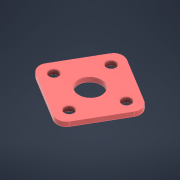
# Autodesk Inventor part: motor bracket n 20
Saved by Autodesk Inventor 2021 (Build 250183000, 183)
## iProperties
Created: 2021-01-01
Part Number: motor bracket n 20
Material: Steel, Mild
Document SubType Name: Modeling
Designer: Vikki
Density: 7.85 g/cm^3
Appearance: Smooth - Red
Author: Vikki
Autodesk Inventor part; units mm, degrees
ref_plane "YZ Plane" through (0, 0, 0) normal (1, 0, 0) x (0, 1, 0)
ref_plane "XZ Plane" through (0, 0, 0) normal (0, 1, 0) x (-1, 0, 0)
ref_plane "XY Plane" through (0, 0, 0) normal (0, 0, 1) x (1, 0, 0)
ref_plane "Work Plane1" through (16.343721, 23.98815, 28.390628) normal (0.0633212, 0.9973467, 0.0359151) x (-0.8897935, 0.0401224, 0.4545962)
sketch "Sketch1" plane through (16.343721, 23.98815, 28.390628) normal (0.0633212, 0.9973467, 0.0359151) x (-0.8897935, 0.0401224, 0.4545962)
  circle A0 centre (9.859, 0) radius 11 construction
  line L0 (12.200549, 7.380964) -> (2.137484, 0.843784)
  line L1 (13.972533, 19.366952) -> (-9.507952, 4.113533)
  line L2 (-9.507952, 4.113533) -> (5.745467, -19.366952)
  line L3 (5.745467, -19.366952) -> (29.225952, -4.113533)
  line L4 (29.225952, -4.113533) -> (13.972533, 19.366952)
  line L5 (13.972533, 19.366952) -> (5.745467, -19.366952) construction
  line L6 (-9.507952, 4.113533) -> (29.225952, -4.113533) construction
  circle A1 centre (9.859, 0) radius 9.5
  circle A2 centre (9.859, 0) radius 9.5
  circle A3 centre (9.859, 0) radius 9.5
  circle A4 centre (9.859, 0) radius 9.5
  point P0 (0.673802, -31.196325)
  dimension "d0" = 28
  dimension "d1" = 28
  dimension "d26" = 19
  constraints: 12 end point, 3 parallel, 2 midpoint, 1 centre point, 1 coincident, 1 perpendicular
  measures "d0" distance of L3.end L1.start
  measures "d1" distance of L2.end L3.end
  measures "d26" diameter of A4
extrude "Extrusion1" add sketch "Sketch1" against normal blind 2
sketch "Sketch2" plane through (16.343721, 23.98815, 28.390628) normal (0.0633212, 0.9973467, 0.0359151) x (0.8897935, -0.0401224, -0.4545962)
  line L0 (-29.225952, 4.113533) -> (-5.745467, 19.366952)
  line L1 (-29.225952, 4.113533) -> (-5.745467, 19.366952)
  line L2 (-5.745467, 19.366952) -> (-6.834997, 21.04413)
  line L3 (-6.834997, 21.04413) -> (-30.315482, 5.790711)
  line L4 (-30.315482, 5.790711) -> (-29.225952, 4.113533)
  point P0 (-0.673802, 31.196325)
  dimension "d4" = 2
  constraints: 8 end point, 3 equal length, 1 perpendicular
  measures "d4" distance of L0.end L2.end
extrude "Extrusion2" add sketch "Sketch2" against normal blind 65
ref_plane "Work Plane2" through (6.048334, 1.450993, 31.990123) normal (0.0633212, 0.9973467, 0.0359151) x (-0.4999648, 0.0005557, 0.8660455)
sketch "Sketch3" plane through (6.048334, 1.450993, 31.990123) normal (0.0633212, 0.9973467, 0.0359151) x (-0.4999648, 0.0005557, 0.8660455)
  circle A0 centre (-3, 2) radius 0.5
  circle A1 centre (3, -2) radius 0.5
  circle A2 centre (0, 0) radius 1.5
  circle A3 centre (0, 0) radius 2
  line L0 (-5, -13.914) -> (5, -13.914)
  line L1 (5, -13.914) -> (5, 13.913999)
  line L2 (5, 13.913999) -> (-5, 13.913999)
  line L3 (-5, 13.913999) -> (-5, -13.914)
  line L4 (-5, -13.914) -> (5, 13.913999) construction
  line L5 (5, -13.914) -> (-5, 13.913999) construction
  line L6 (14.015513, -13.914) -> (-13.984487, -13.914)
  line L7 (-13.984487, -13.914) -> (14.015513, -13.914)
  line L8 (-5, 4) -> (5, 4)
  line L9 (-13.984487, -13.914) -> (14.015513, -13.914)
  line L10 (14.015513, -13.914) -> (14.015513, -5.914)
  line L11 (14.015513, -5.914) -> (-13.984487, -5.914)
  line L12 (-13.984487, -5.914) -> (-13.984487, -13.914)
  point P0 (-24.681756, -21.071113)
  point P1 (5, -5.914)
  point P2 (5, -13.914)
  point P3 (-5, -13.914)
  point P4 (-5, -5.914)
  dimension "d8" = 10
  dimension "d9" = 2
  dimension "d17" = 8
  constraints: 22 end point, 4 parallel, 3 perpendicular, 2 horizontal, 2 midpoint, 2 point on line, 1 collinear
  measures "d8" distance of L1.end L2.end
  measures "d9" distance from line of L8 A0.centre
  measures "d17" distance of L6.start L10.end
extrude "Extrusion3" add sketch "Sketch3" along normal blind 2 contours L3 L11 L1 L0 | L6 L12 L11 L3 | L1 L11 L10 L6 | L3 L8 L1 L11
sketch "Sketch4" plane through (12.227841, -40.839389, 26.056144) normal (-0.0633212, -0.9973467, -0.0359151) x (0.8897935, -0.0401224, -0.4545962)
  line L0 (-29.225952, -4.113533) -> (-5.745467, -19.366952)
  line L1 (-5.745467, -19.366952) -> (9.507952, 4.113533)
  line L2 (9.507952, 4.113533) -> (-13.972533, 19.366952)
  line L3 (-13.972533, 19.366952) -> (-29.225952, -4.113533)
  circle A0 centre (-9.859, 0) radius 5
  point P0 (-0.673802, -31.196325)
  dimension "d12" = 10
  constraints: 1 centre point
  measures "d12" diameter of A0
extrude "Extrusion4" add sketch "Sketch4" against normal blind 2
sketch "Sketch5" plane through (16.343721, 23.98815, 28.390628) normal (0.0633212, 0.9973467, 0.0359151) x (0.8897935, -0.0401224, -0.4545962)
  line L0 (-29.225952, 4.113533) -> (-5.745467, 19.366952)
  line L1 (-5.745467, 19.366952) -> (-29.225952, 4.113533)
  line L2 (-29.225952, 4.113533) -> (-30.315482, 5.790711)
  line L3 (-30.315482, 5.790711) -> (-6.834997, 21.04413)
  line L4 (-6.834997, 21.04413) -> (-5.745467, 19.366952)
  line L5 (-30.315482, 5.790711) -> (-13.972533, -19.366952)
  point P0 (-0.673802, 31.196325)
  constraints: 8 end point, 2 parallel, 2 perpendicular
extrude "Extrusion5" cut sketch "Sketch5" against normal up to surface (65 mm away)
sketch "Sketch6" plane through (16.343721, 23.98815, 28.390628) normal (0.0633212, 0.9973467, 0.0359151) x (0.8897935, -0.0401224, -0.4545962)
  circle A0 centre (-12.45606, -12.227235) radius 2
  line L0 (-13.972533, -19.366952) -> (-29.225952, 4.113533)
  circle A1 centre (-22.086235, 2.59706) radius 2
  circle A2 centre (-7.26194, 12.227235) radius 2
  circle A3 centre (2.368235, -2.59706) radius 2
  circle A4 centre (-9.859, 0) radius 12.5
  circle A5 centre (-9.859, 0) radius 9.5
  line L1 (-13.972533, -19.366952) -> (9.507952, -4.113533)
  line L2 (9.507952, -4.113533) -> (-9.859, 0) construction
  point P0 (-0.673802, 31.196325)
  dimension "d35" = 25
  dimension "d19" = 4
  dimension "d22" = 360
  constraints: 4 centre point, 2 coincident, 2 end point, 1 point on line, 12 other
  measures "d19" diameter of A0
extrude "Extrusion6" add sketch "Sketch6" against normal up to surface (65 mm away) contours A0 A4 | A4 A0 | A4 A1 | A1 A4 | A4 A3 | A3 A4 | A4 A2 | A2 A4
sketch "Sketch7" plane through (6.174976, 3.445687, 32.061954) normal (0.0633212, 0.9973467, 0.0359151) x (0.8637277, -0.0727954, 0.4986734)
  line L0 (14.086, 13.984487) -> (-13.914, 13.984487)
  line L1 (14.086, -14.015513) -> (14.086, 13.984487)
  line L2 (-13.914, -14.015513) -> (14.086, -14.015513)
  line L3 (4.086, 13.984487) -> (4.086, -14.015513)
  line L4 (4, 5) -> (4.086, 5)
  line L5 (-5.914, -5) -> (4, -5)
  line L6 (4, -5) -> (4.086, -5)
  line L7 (4, -5) -> (4, 5)
  circle A0 centre (8.924835, 8.823322) radius 2
  circle A1 centre (8.924835, 8.823322) radius 2
  line L8 (-3.914, 13.984487) -> (-3.914, -14.015513)
  line L9 (-13.914, -14.015513) -> (-13.914, 13.984487)
  point P0 (-21.071113, 24.681756)
  dimension "d36" = 10
  dimension "d37" = 10
  constraints: 8 end point, 6 point on line, 4 perpendicular, 1 coincident
  measures "d36" distance between parallel lines of L1 L3
  measures "d37" distance between parallel lines of L8 L9
extrude "Extrusion7" add sketch "Sketch7" against normal up to surface (2 mm away) contours L1 L2 L3 L0 | L8 L2 L9 L0 | L3 L6 L7 L4
sketch "Sketch9" plane through (16.343721, 23.98815, 28.390628) normal (0.0633212, 0.9973467, 0.0359151) x (0.8897935, -0.0401224, -0.4545962)
  circle A0 centre (-9.859, 0) radius 9.5 projected
  circle A1 centre (-9.859, 0) radius 6.5
  point P0 (-0.673802, 31.196325)
  dimension "d40" = 13
  constraints: 1 centre point, 1 coincident
  measures "d40" diameter of A1
extrude "Extrusion8" add sketch "Sketch9" against normal up to surface (2 mm away)
thread "Thread5" size "M4x0.7" class "6g" standard "ANSI Metric M Profile" full length
thread "Thread6" size "M4x0.7" class "6g" standard "ANSI Metric M Profile" full length
thread "Thread7" size "M4x0.7" class "6g" standard "ANSI Metric M Profile" full length
thread "Thread8" size "M4x0.7" class "6g" standard "ANSI Metric M Profile" full length
sketch "Sketch10" plane through (6.174976, 3.445687, 32.061954) normal (0.0633212, 0.9973467, 0.0359151) x (0.8637277, -0.0727954, 0.4986734)
  circle A0 centre (8.924835, -8.854348) radius 2
  circle A1 centre (8.924835, 8.823322) radius 2
  circle A2 centre (-8.752834, -8.854348) radius 2
  circle A3 centre (-8.752834, 8.823322) radius 2
  line L0 (-3.914, -5) -> (4.086, -5)
  line L1 (4.086, -5) -> (4.086, -14.015513)
  line L2 (4.086, -14.015513) -> (14.086, -14.015513)
  line L3 (14.086, -14.015513) -> (14.086, 13.984487)
  line L4 (14.086, 13.984487) -> (4.086, 13.984487)
  line L5 (4.086, 13.984487) -> (4.086, 5)
  line L6 (4.086, 5) -> (-3.914, 5)
  line L7 (-3.914, 5) -> (-3.914, 13.984487)
  line L8 (-3.914, 13.984487) -> (-13.914, 13.984487)
  line L9 (-13.914, -14.015513) -> (-13.914, 13.984487)
  line L10 (-13.914, -14.015513) -> (-3.914, -14.015513)
  line L11 (-3.914, -14.015513) -> (-3.914, -5)
  circle A4 centre (-2, -3) radius 0.5
  circle A5 centre (2, 3) radius 0.5
  circle A6 centre (0, 0) radius 2
  line L12 (4.086, 13.984487) -> (4.086, 5)
  line L13 (-3.914, 13.984487) -> (-13.914, 13.984487)
  line L14 (4.086, 13.984487) -> (-3.914, 13.984487)
  line L15 (-13.914, -14.015513) -> (-3.914, -14.015513)
  line L16 (4.086, -14.015513) -> (-3.914, -14.015513)
  point P0 (-21.071113, 24.681756)
  constraints: 4 end point, 1 collinear, 1 horizontal
extrude "Extrusion9" add sketch "Sketch10" against normal up to surface (2 mm away) contours L0 L1 L16 L11 | L14 L5 L6 L7
fillet "Fillet1" radius 4 12 edges at (8.6114, -40.4578, 49.68) (22.6104, -40.4734, 25.4307) (-1.574, -38.4351, 11.4679) (-15.573, -38.4196, 35.7171) (-12.9135, 3.469, 37.2256) (1.0855, 3.4534, 12.9763) (25.2699, 1.4152, 26.9392) (11.2709, 1.4307, 51.1884) (12.6006, 22.375, 51.9426) (26.5996, 22.3595, 27.6934) (2.4152, 24.3977, 13.7305) (-11.5838, 24.4133, 37.9798)
sketch "Sketch17" plane through (12.354484, -38.844695, 26.127975) normal (0.0633212, 0.9973467, 0.0359151) x (0.8897935, -0.0401224, -0.4545962)
  circle A0 centre (-7.26194, 12.227235) radius 2
  circle A1 centre (-22.086235, 2.59706) radius 2
  circle A2 centre (-12.45606, -12.227235) radius 2
  circle A3 centre (2.368235, -2.59706) radius 2
  point P0 (-0.673802, 31.196325)
extrude "Extrusion15" cut sketch "Sketch17" against normal up to surface (2 mm away)
sketch "Sketch18" plane through (16.343721, 23.98815, 28.390628) normal (0.0633212, 0.9973467, 0.0359151) x (0.8897935, -0.0401224, -0.4545962)
  circle A0 centre (-9.859, 0) radius 6.5 construction
  arc A1 (-25.871597, 6.292593) -> (-27.046893, 0.759178) centre (-23.692537, 2.938238) ccw
  line L0 (-27.046893, 0.759178) -> (-16.151593, -16.012597)
  arc A2 (-16.151593, -16.012597) -> (-10.618178, -17.187893) centre (-12.797238, -13.833537) ccw
  line L1 (-10.618178, -17.187893) -> (6.153597, -6.292593)
  arc A3 (6.153597, -6.292593) -> (7.328893, -0.759178) centre (3.974537, -2.938238) ccw
  line L2 (7.328893, -0.759178) -> (-3.566407, 16.012597)
  arc A4 (-3.566407, 16.012597) -> (-9.099822, 17.187893) centre (-6.920762, 13.833537) ccw
  line L3 (-9.099822, 17.187893) -> (-25.871597, 6.292593)
  point P0 (-0.673802, 31.196325)
extrude "Extrusion16" cut sketch "Sketch18" against normal up to surface (63 mm away)
body "Solid1"
